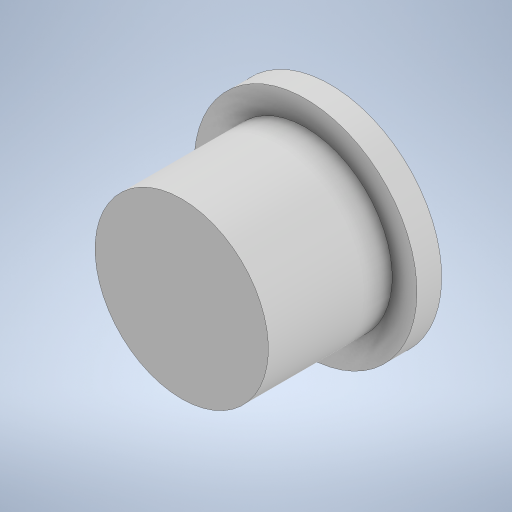
# Autodesk Inventor part: Деталь4
Saved by Autodesk Inventor 2024 (Build 280153000, 153)
## iProperties
Created: 2023-10-26
Part Number: Деталь4
Material: Типовые
Document SubType Name: Sheet Metal
Designer: Elisey
Density: 1 g/cm^3
Sheet Metal Rule: По умолчанию_мм
Appearance: По умолчанию
Author: Elisey
Autodesk Inventor part; units mm, degrees
ref_plane "YZ Plane" through (0, 0, 0) normal (1, 0, 0) x (0, 1, 0)
ref_plane "XZ Plane" through (0, 0, 0) normal (0, 1, 0) x (-1, 0, 0)
ref_plane "XY Plane" through (0, 0, 0) normal (0, 0, 1) x (1, 0, 0)
sketch "Эскиз1" plane through (0, 0, 0) normal (1, 0, 0) x (0, 1, 0)
  line L0 (-0.0944, -29.3854) -> (-9.0944, -29.3854)
  line L1 (-9.0944, -29.3854) -> (-9.0944, -27.3854)
  line L2 (-9.0944, -27.3854) -> (-7.0944, -27.3854)
  line L3 (-7.0944, -27.3854) -> (-7.0944, -17.3854)
  line L4 (-7.0944, -17.3854) -> (-0.0944, -17.3854)
  line L5 (-0.0944, -17.3854) -> (-0.0944, -19.3854)
  line L6 (-0.0944, -19.3854) -> (-4.0944, -19.3854)
  line L7 (-4.0944, -19.3854) -> (-4.0944, -20.8854)
  line L8 (-4.0944, -20.8854) -> (-3.0944, -20.8854)
  line L9 (-3.0944, -20.8854) -> (-3.0944, -29.3854)
  line L10 (-0.0944, -15.3854) -> (-0.0944, -31.3854)
  point P0 (0, 0)
  point P1 (-105.6045, -1.7251)
  constraints: 22 end point, 4 perpendicular, 1 parallel, 1 point on line
revolve "Вращение1" add sketch "Эскиз1" angle 360 about axis through (0, -0.0944, -15.3854) along (0, 0, -1) contours L0 L1 L2 L3 L4 L5 L6 L7 L8 L9
equation "\"Радиус_гибки\" = Толщина"
equation "\"Ширина_просечки\" = Толщина"
equation "\"Глубина_просечки\" = 0.5 * Толщина"
equation "\"Размер_просечки\" = 4 * Толщина"
equation "\"Мин_остаток\" = 2 * Толщина"
equation "\"Радиус_перехода\" = Радиус_гибки"
equation "\"Радиус_Якоби\" = Радиус_гибки"
equation "\"Размер_зазора\" = Толщина"
equation "\"Толщина\" = 0.5"
